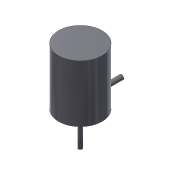
# Autodesk Inventor part: P01 - Fan Motor
Saved by Autodesk Inventor 2016 (Build 200138000, 138)
## iProperties
Created: 2016-12-26
Part Number: P01 - Fan Motor
Material: SAE 1020
Document SubType Name: Modeling
Designer: Fernando
Stock Number: 0
Mass: 5955.75 g
Surface Area: 497.431 cm^2
Volume: 756.766 cm^3
Density: 7.87 g/cm^3
Appearance: Steel - Polished
SurfaceArea_m2: .05
Author: Fernando
Autodesk Inventor part; units mm, degrees
ref_plane "YZ Plane" through (0, 0, 0) normal (1, 0, 0) x (0, 1, 0)
ref_plane "XZ Plane" through (0, 0, 0) normal (0, 1, 0) x (-1, 0, 0)
sketch "Sketch2" plane through (0, 0, 0) normal (0, 0, 1) x (1, 0, 0)
  circle A0 centre (0, 0) radius 45
  dimension "d11" = 90
  constraints: 1 centre point, 1 coincident
  measures "d11" diameter of A0
extrude "Extrusion2" add sketch "Sketch2" along normal blind 118
sketch "Sketch3" plane through (0, 0, 0) normal (0, 0, -1) x (-1, 0, 0)
  circle A0 centre (0, 0) radius 4
  dimension "d14" = 8
  constraints: 1 centre point, 1 coincident
  measures "d14" diameter of A0
extrude "Extrusion3" add sketch "Sketch3" along normal blind 70
thread "Thread1" size "M8x1.25" class "6g" standard "ANSI Metric M Profile" length 17
sketch "Sketch4" plane through (0, 0, -70) normal (0, 0, -1) x (-1, 0, 0)
  line L0 (3.4641, 2) -> (-3.4641, 2)
  arc A0 (3.4641, 2) -> (-3.4641, 2) centre (0, 0) ccw
  circle A1 centre (0, 0) radius 4 projected
  dimension "d19" = 2
  constraints: 2 end point, 2 point on circle, 1 centre point, 1 coincident, 1 concentric, 1 horizontal
  measures "d19" distance from line of point (0, 0) L0
extrude "Extrusion4" cut sketch "Sketch4" against normal blind 17 contours L0 A0
ref_plane "Work Plane1" through (0, 0, -28) normal (0, 0, -1) x (-1, 0, 0)
sketch "Sketch5" plane through (0, 0, -28) normal (0, 0, -1) x (-1, 0, 0)
  circle A0 centre (0, 0) radius 4 projected
  circle A1 centre (0, 0) radius 5.5
  dimension "d23" = 1.5
  constraints: 1 centre point, 1 coincident
  measures "d23" radial gap between concentric circles of A1 A0
extrude "Extrusion5" add sketch "Sketch5" against normal blind 1
sketch "Sketch6" plane through (0, 0, 0) normal (0, 0, -1) x (-1, 0, 0)
  circle A0 centre (0, 0) radius 26 construction
  point P0 (0, -26)
  point P1 (-26, 0)
  point P2 (0, 26)
  point P3 (26, 0)
  dimension "d26" = 52
  constraints: 4 point on circle, 2 horizontal alignment, 2 vertical alignment, 1 centre point, 1 coincident
  measures "d26" diameter of A0
hole "Hole1" at (0, -26, 0) at (26, 0, 0) at (0, 26, 0) at (-26, 0, 0) direction (0, 0, 1) diameter 3.242 depth 15 tip angle 118 thread size "M4x0.7" class "6H" standard "ANSI Metric M Profile"
sketch "Sketch7" plane through (0, 0, 0) normal (0, 1, 0) x (-1, 0, 0)
  circle A0 centre (0, 14.6614) radius 5
  point P0 (0, 0)
  dimension "d34" = 10
  constraints: 1 centre point, 1 vertical alignment
  measures "d34" diameter of A0
extrude "Extrusion6" add sketch "Sketch7" along normal blind 85
body "Solid2"
